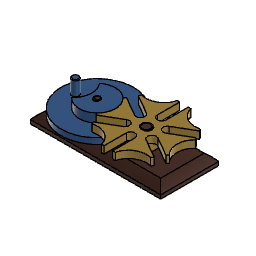
Geneva Mechanism (Autodesk Fusion 360 design; units mm, degrees)
Autodesk Fusion 360 part; units mm, degrees
sketch "Sketch1" plane through (0, 0, 0) normal (0, 0, 1) x (1, 0, 0)
  line L0 (0, 0) -> (180, 0)
  line L1 (180, 0) -> (180, 80)
  line L2 (180, 80) -> (0, 80)
  line L3 (0, 80) -> (0, 0)
  line L4 (90, 80) -> (90, 0) construction
  line L5 (0, 40) -> (180, 40) construction
  circle A0 centre (52.5, 40) radius 7.5
  line L6 (60, 40) -> (90, 40)
  circle A1 centre (120, 40) radius 7.5
  circle A2 centre (52.5, 40) radius 50
  circle A3 centre (52.5, 40) radius 25
  line L7 (70, 68.8675) -> (70, 11.1325) construction
  line L8 (70, 11.1325) -> (120, -17.735) construction
  line L9 (120, -17.735) -> (170, 11.1325) construction
  line L10 (170, 11.1325) -> (170, 68.8675) construction
  line L11 (170, 68.8675) -> (120, 97.735) construction
  line L12 (120, 97.735) -> (70, 68.8675) construction
  circle A4 centre (87.5, 40) radius 25
  line L13 (120, 40) -> (70, 11.1325) construction
  line L14 (98.3234, 34.4132) -> (67, 16.3286)
  line L15 (104.3234, 24.0209) -> (73, 5.9363)
  line L16 (120, 40) -> (70, 68.8675) construction
  line L17 (104.3234, 55.9791) -> (73, 74.0637)
  line L18 (67, 63.6714) -> (98.3234, 45.5868)
  line L19 (170, 40) -> (187.5, 40) construction
  line L20 (120, 40) -> (145, -3.3013) construction
  line L21 (145, -3.3013) -> (153.75, -18.4567) construction
  line L22 (120, 40) -> (145, 83.3013) construction
  line L23 (145, 83.3013) -> (153.75, 98.4567) construction
  circle A5 centre (187.5, 40) radius 25
  circle A6 centre (153.75, 98.4567) radius 25
  circle A7 centre (153.75, -18.4567) radius 25
  line L24 (52.5, 40) -> (70, 11.1325) construction
  circle A8 centre (85, 40) radius 5
  line L25 (95, -3.3013) -> (86.25, -18.4567) construction
  circle A9 centre (86.25, -18.4567) radius 25
  line L26 (120, 40) -> (95, 83.3013) construction
  line L27 (95, 83.3013) -> (86.25, 98.4567) construction
  circle A10 centre (86.25, 98.4567) radius 25
  arc A11 (67, 16.3286) -> (73, 5.9363) centre (70, 11.1325) ccw
  arc A12 (104.3234, 24.0209) -> (98.3234, 34.4132) centre (101.3234, 29.2171) ccw
  arc A13 (73, 74.0637) -> (67, 63.6714) centre (70, 68.8675) ccw
  arc A14 (98.3234, 45.5868) -> (104.3234, 55.9791) centre (101.3234, 50.7829) ccw
  circle A15 centre (120, 97.735) radius 6
  circle A16 centre (170, 68.8675) radius 6
  circle A17 centre (170, 11.1325) radius 6
  circle A18 centre (138.6685, 29.2222) radius 6
  circle A19 centre (138.6767, 50.783) radius 6
  circle A20 centre (120, 61.566) radius 6
  line L28 (120, 67.566) -> (120, 97.735) construction
  line L29 (143.8729, 53.783) -> (170, 68.8675) construction
  line L30 (120, 40) -> (126.4952, 36.25) construction
  line L31 (143.8644, 26.2219) -> (170, 11.1325) construction
  line L32 (70, 22.1464) -> (71.7692, 19.0821)
  line L33 (79.5384, 5.6255) -> (77.7692, 8.6898)
  line L34 (114, 18.434) -> (114, -17.735)
  line L35 (126, 18.434) -> (126, -17.735)
  line L36 (120, 40) -> (120, 24.434) construction
  line L37 (120, 12.434) -> (120, -17.735) construction
  arc A21 (126, 18.434) -> (114, 18.434) centre (120, 18.434) ccw
  arc A22 (114, -17.735) -> (126, -17.735) centre (120, -17.735) ccw
  line L38 (173.0001, 16.3286) -> (141.6685, 34.4183)
  line L39 (135.6684, 24.0261) -> (166.9999, 5.9364)
  line L40 (167, 74.0637) -> (135.6767, 55.9792)
  line L41 (173, 63.6714) -> (141.6767, 45.5868)
  line L42 (114, 97.735) -> (114, 61.566)
  line L43 (126, 97.735) -> (126, 61.566)
  line L44 (110.4616, -12.2281) -> (114, -12.2281)
  line L45 (129.5384, -12.2281) -> (126, -12.2281)
  line L46 (160.4616, 5.6255) -> (162.2309, 8.6899)
  line L47 (170, 22.1464) -> (168.2308, 19.0822)
  line L48 (170, 57.8536) -> (168.2308, 60.9179)
  line L49 (160.4616, 74.3745) -> (162.2308, 71.3102)
  line L50 (129.5384, 92.2281) -> (126, 92.2281)
  line L51 (110.4616, 92.2281) -> (114, 92.2281)
  line L52 (70, 57.8536) -> (71.7692, 60.9179)
  line L53 (79.5384, 74.3745) -> (77.7692, 71.3102)
  circle A23 centre (120, 40) radius 12.5
  circle A24 centre (52.5, 40) radius 5
  circle A25 centre (52.5, 40) radius 12.5
  circle A26 centre (52.5, 40) radius 4
  circle A27 centre (120, 40) radius 6.5
  point P0 (120, 40)
  point P1 (70, 57.8536)
  point P2 (70, 40)
  point P3 (77.5, 40)
  point P4 (102.5, 40)
  point P5 (65.46, 18.6215)
  dimension "d2" = 30
  dimension "d4" = 30
  dimension "d5" = 100
  dimension "d6" = 50
  dimension "d8" = 50
  dimension "d10" = 180
  dimension "d11" = 80
  dimension "d15" = 12
  dimension "d19" = 17.5
  dimension "d26" = 7.4891
  dimension "d27" = 10
  dimension "d28" = 7.5
  dimension "d48" = 25
  dimension "d61" = -1
  dimension "d62" = -1
  constraint horizontal L0
  constraint vertical L1
  constraint horizontal L2
  constraint vertical L3
  constraint coincident L0.start L3.end
  constraint midpoint L2 L4.start
  constraint midpoint L0 L4.end
  constraint midpoint L3 L5.start
  constraint midpoint L1 L5.end
  constraint coincident L5 A0.centre
  constraint coincident L5 L6.start
  constraint coincident A0 L6.start
  constraint midpoint L5 L6.end
  constraint perpendicular L4 L6
  constraint coincident L5 P0
  constraint concentric A0 A2
  constraint concentric A2 A3
  constraint coincident P0 A1.centre
  constraint parallel L4 L7
  constraint coincident L5 A4.centre
  constraint coincident A3 P1
  constraint coincident L7 P1
  constraint midpoint L7 P2
  constraint coincident L5 P3
  constraint coincident A3 P3
  constraint coincident A4 P1
  constraint coincident A2 P4
  constraint coincident L5 P4
  constraint coincident L7.end L8.start
  constraint coincident L13 A12.centre
  constraint coincident A2 A12.centre
  constraint tangent L14 A11
  constraint tangent L15 A11
  constraint tangent L14 A12
  constraint tangent L15 A12
  constraint coincident L7.start L12.end
  constraint coincident L16 A14.centre
  constraint coincident A2 A14.centre
  constraint parallel L16 L17
  constraint tangent L18 A14
  constraint tangent L18 A13
  constraint tangent L17 A13
  constraint tangent L17 A14
  constraint midpoint L10 L19.start
  constraint perpendicular L10 L19
  constraint midpoint L9 L20.end
  constraint perpendicular L9 L21
  constraint midpoint L11 L22.end
  constraint perpendicular L11 L23
  constraint coincident L19.end A5.centre
  constraint coincident L23.end A6.centre
  constraint coincident L21.end A7.centre
  constraint coincident A0.centre A2.centre
  constraint coincident L24 P5
  constraint coincident A3 P5
  constraint coincident L5 A8.centre
  constraint midpoint L8 L25.start
  constraint perpendicular L8 L25
  constraint coincident L25.end A9.centre
  constraint midpoint L12 L26.end
  constraint perpendicular L12 L27
  constraint coincident L27.end A10.centre
  constraint coincident L11.end L12.start
  constraint coincident L10.end L11.start
  constraint coincident L8.end L9.start
  constraint coincident L9.end L10.start
  constraint coincident A20 L28.start
  constraint coincident A19 L29.start
  constraint coincident A1 L30.end
  constraint collinear L30 L31
  constraint coincident A3 L32.start
  constraint coincident A4 L32.start
  constraint coincident L14 L32.end
  constraint perpendicular L14 L32
  constraint coincident A9 L33.start
  constraint coincident L8 L33.start
  constraint coincident L15 L33.end
  constraint perpendicular L15 L33
  constraint tangent L34 A22
  constraint tangent L35 A22
  constraint tangent L34 A21
  constraint tangent L35 A21
  constraint coincident L36.end A21
  constraint collinear L36 L37
  constraint coincident A18 L31.start
  constraint coincident A17 L38.start
  constraint coincident A18 L38.end
  constraint tangent A18 L38
  constraint coincident A18 L39.start
  constraint coincident A17 L39.end
  constraint tangent A17 L39
  constraint coincident A16 L40.start
  constraint coincident A19 L40.end
  constraint tangent A19 L40
  constraint coincident A16 L41.start
  constraint coincident A19 L41.end
  constraint tangent A19 L41
  constraint coincident A15 L42.start
  constraint coincident A20 L42.end
  constraint tangent A20 L42
  constraint coincident A15 L43.start
  constraint coincident A20 L43.end
  constraint tangent A20 L43
  constraint tangent A15 L42
  constraint tangent A15 L43
  constraint tangent A16 L40
  constraint tangent A16 L41
  constraint tangent A17 L38
  constraint tangent A18 L39
  constraint coincident A9 L44.start
  constraint coincident L8 L44.start
  constraint coincident L34 L44.end
  constraint perpendicular L34 L44
  constraint coincident L9 L45.start
  constraint coincident A7 L45.start
  constraint coincident L35 L45.end
  constraint perpendicular L35 L45
  constraint coincident A7 L46.start
  constraint coincident L9 L46.start
  constraint coincident L39 L46.end
  constraint perpendicular L39 L46
  constraint coincident A5 L47.start
  constraint coincident L10 L47.start
  constraint coincident L38 L47.end
  constraint perpendicular L38 L47
  constraint coincident L10 L48.start
  constraint coincident A5 L48.start
  constraint coincident L41 L48.end
  constraint perpendicular L41 L48
  constraint coincident A6 L49.start
  constraint coincident L11 L49.start
  constraint coincident L40 L49.end
  constraint perpendicular L40 L49
  constraint coincident A6 L50.start
  constraint coincident L11 L50.start
  constraint coincident L43 L50.end
  constraint perpendicular L43 L50
  constraint coincident L12 L51.start
  constraint coincident A10 L51.start
  constraint coincident L42 L51.end
  constraint perpendicular L42 L51
  constraint coincident P1 L52.start
  constraint coincident L18 L52.end
  constraint perpendicular L18 L52
  constraint coincident L12 L53.start
  constraint coincident A10 L53.start
  constraint coincident L17 L53.end
  constraint perpendicular L17 L53
  constraint concentric A2 A24
  constraint concentric A0 A25
  measures "d2" distance of L6.start L6.end
  measures "d4" distance of L6.end P0
  measures "d5" diameter of A2
  measures "d6" diameter of A3
  measures "d8" diameter of A4
  measures "d10" distance of L0.start L0.end
  measures "d11" distance of L0.start L2.end
  measures "d15" diameter of A11
  measures "d19" distance of A0.centre P2
  measures "d26" vertical distance of L7.end P5
  measures "d27" diameter of A8
  measures "d28" distance of P3 A8.centre
  measures "d48" diameter of A23
extrude "Extrude4" add sketch "Sketch1" along normal blind 20 contours A3 A4 A25 | A4 A25 | A0 | L6 A8 | L6 A8 makes body 1 at (69.1068, 21.3127, 13.3333) makes body 2 at (89.9752, 40.4978, 13.3333)
extrude "Extrude1" add sketch "Sketch1" along normal blind 10 separate body contours A2 A4 L15 A9 L33 | L0 L2 A2 A4 A5 A6 A7 A9 A10 A18 A19 A20 L34 L35 A21 L38 L39 L40 L41 L42 L43 L46 L47 L48 L49 A23 | L0 A9 L34 L44 | A2 A4 L17 A10 L53 | A2 A4 L15 | A2 A4 L15 L17 A12 A14 A23 | L2 A10 L42 L51 | L0 A7 L35 L45 | A4 A23 | A4 A23 | A4 L14 L32 | A2 A3 A4 L14 L18 A12 A14 | A2 A4 L17 | L2 A6 L43 L50 | A4 L18 L52 | L6 A8 | L6 A8 makes body 3
extrude "Extrude2" add sketch "Sketch1" against normal blind 12 contours A4 A23 | A4 A23 bodies 3
copy_body "Body->Comp1" bodies 3 removing the originals makes body 4 in component "Hexagon"
extrude "Extrude3" add sketch "Sketch1" along normal blind 10 separate body contours L0 L2 A2 A3 L14 L15 L17 L18 A9 A10 A11 A13 L32 L33 L52 L53 | L0 A2 A9 | L0 A2 A9 | L0 A2 A9 | L2 A2 A10 | A2 A4 L15 A9 L33 | L2 A2 A10 | L2 A2 A10 | A4 L14 L15 A11 | A2 A4 L17 A10 L53 | A2 A4 L15 | A2 A4 L14 L15 A12 | A4 L17 L18 A13 | A4 L14 L32 | A2 A3 A4 L14 L18 A12 A14 | A2 A4 L17 | A2 A4 L17 L18 A14 | L6 A3 A4 A25 | A3 A4 A25 | A4 L18 L52 | L6 A3 A4 A25 | A4 A25 | L6 A4 A25 | L6 A4 A25 | A0 | L6 A8 | L6 A8 picked at (40.1327, -1.2898) picked at (81.6151, 3.9769) picked at (71.9676, -3.565) picked at (40.1327, 81.2898) picked at (71.9676, 83.565) picked at (81.6151, 76.0231) makes body 5
combine "Combine1" operation add target body 1 tool bodies 2 5
extrude "Extrude5" add sketch "Sketch1" against normal blind 2 contours A4 A25 | L6 A4 A25 | L6 A4 A25 bodies 1
copy_body "Body->Comp2" bodies 1 removing the originals makes body 6 in component "Circle"
extrude "Extrude6" add sketch "Sketch1" along normal blind 24 separate body contours A26 | A27 makes body 7 at (56.495, 39.8006, 16) makes body 8 at (126.4919, 39.676, 16)
extrude "Extrude7" add sketch "Sketch1" against normal blind 15 contours L0 L2 L3 A2 | L0 L2 A2 A3 L14 L15 L17 L18 A9 A10 A11 A13 L32 L33 L52 L53 | L0 A2 A9 | L0 A2 A9 | A2 A4 L15 A9 L33 | L2 A2 A10 | L0 L2 A2 A4 A5 A6 A7 A9 A10 A18 A19 A20 L34 L35 A21 L38 L39 L40 L41 L42 L43 L46 L47 L48 L49 A23 | A4 L14 L15 A11 | L2 A2 A10 | A2 A4 L17 A10 L53 | L0 L34 L35 A21 | A2 A4 L15 | A2 A4 L15 L17 A12 A14 A23 | A2 A4 L14 L15 A12 | A4 L17 L18 A13 | A2 L15 A12 | A4 A23 | A1 | A4 A23 | A4 L14 L32 | A2 A3 A4 L14 L18 A12 A14 | L2 A20 L42 L43 | A2 A4 L17 | A2 A4 L17 L18 A14 | L0 A7 | L6 A3 A4 A25 | A3 A4 A25 | A20 | A2 L17 A14 | A4 L18 L52 | L0 L1 A5 A7 A17 L38 L39 L46 L47 | L6 A3 A4 A25 | A4 A25 | L6 A4 A25 | L2 A6 | A17 A18 L38 L39 | L6 A4 A25 | L1 L2 A5 A6 A16 L40 L41 L48 L49 | L1 A5 | A18 | A17 | A16 A19 L40 L41 | A16 | A19 | A0 | L6 A8 | L6 A8 | A24 | A26 | A27 picked at (81.6151, 3.9769) picked at (90.189, 0.6547) picked at (81.6151, 76.0231) picked at (95.4497, 79.3605) picked at (155.593, 3.5272) picked at (158.6135, 79.3853) picked at (177.4057, 46.5949) bodies 7 8
copy_body "Body->Comp3" bodies 7 removing the originals makes body 9 in component "Base"
move_body "Move1" bodies 9 to x (1, 0, 0) y (0, 1, 0) z (0, 0, 1) at (0, 0, 15) in component "Base"
move_body "Move1'" bodies 6 to x (-1, 0, 0) y (0, -1, 0) z (0, 0, 1) at (105, 80, 0) in component "Circle"
fillet "Fillet1" radius 10 tangency weight 0.1 4 edges at (0, 40, 15) (90, 0, 15) (90, 80, 15) (180, 40, 15) on bodies 9 in component "Base"
extrude "Extrude1'" cut 1 faces at (115.1859, 39.9202, 39) faces seen with x (1, 0, 0) y (0, 1, 0) z (0, 0, 1) at (0.5396, -1.5466, -27.0198) along direction (0, 0, -1) blind 2 on bodies 9 bodies 4 in component "Hexagon"
extrude "Extrude1''" cut 1 faces at (115.1859, 39.9202, 39) along direction (0, 0, -1) blind 2 on bodies 9 bodies 9 in component "Base"
extrude "Extrude1'''" cut 1 faces at (51.2702, 39.8013, 39) faces seen with x (1, 0, 0) y (0, 1, 0) z (0, 0, 1) at (0.5396, -1.5466, -17.0198) along direction (0, 0, -1) blind 2 on bodies 9 bodies 6 in component "Circle"
extrude "Extrude2'" cut 1 faces at (51.2702, 39.8013, 39) along direction (0, 0, -1) blind 2 on bodies 9 bodies 9 in component "Base"
fillet "Fillet2" radius 1 2 edges at (113.9399, 42.3505, 37) (48.7707, 41.4465, 37) on bodies 9 in component "Base"
extrude "Extrude2''" add 1 faces at (18.4074, 40.955, 20) along direction (0, 0, 1) blind 8 on bodies 6 bodies 6 in component "Circle"
fillet "Fillet2'" radius 1 1 edges at (24.6616, 41.8081, 28) on bodies 6 in component "Circle"
extrude "Extrude3'" cut 1 faces at (22.1872, 57.0019, 10) along direction (0, 0, -1) blind 2 on bodies 6 bodies 6 in component "Circle"
extrude "Extrude4'" add 1 faces at (41.7411, 40.9936, -2) along direction (0, 0, 1) blind 2 on bodies 6 bodies 6 in component "Circle"
extrude "Extrude5'" cut 1 faces at (41.7411, 40.9936, -2) along direction (0, 0, 1) blind 3 on bodies 6 bodies 6 in component "Circle"
extrude "Extrude6'" add 1 faces at (41.7411, 40.9936, 1) along direction (0, 0, -1) blind 1 on bodies 6 bodies 6 in component "Circle"
extrude "Extrude3''" add sketch "Sketch1" along normal blind 15.8259 contours A4 A25 | L6 A4 A25 | L6 A4 A25 | A0 sketch seen with x (1, 0, 0) y (0, 1, 0) z (0, 0, 1) at (0, 0, 1.1741) bodies 9 in component "Base"
sketch "Hexagon detail" plane through (0, 0, 10) normal (0, 0, 1) x (-1, 0, 0) in component "Hexagon"
  arc A0 (-116.4789, -33.3779) -> (-126.8764, -37.0058) centre (-120.5396, -38.4534) ccw
  arc A1 (-126.8764, -37.0058) -> (-116.4789, -33.3779) centre (-120, -40) ccw
  arc A2 (-79.5384, -74.3745) -> (-110.4616, -92.2281) centre (-86.25, -98.4567) ccw
  line L0 (-79.5384, -74.3745) -> (-77.7692, -71.3102)
  line L1 (-77.7692, -71.3102) -> (-104.3234, -55.9791)
  arc A3 (-98.3234, -45.5868) -> (-104.3234, -55.9791) centre (-101.3234, -50.7829) ccw
  line L2 (-98.3234, -45.5868) -> (-71.7692, -60.9179)
  line L3 (-71.7692, -60.9179) -> (-70, -57.8536)
  arc A4 (-70, -22.1464) -> (-70, -57.8536) centre (-52.5, -40) ccw
  line L4 (-70, -22.1464) -> (-71.7692, -19.0821)
  line L5 (-71.7692, -19.0821) -> (-98.3234, -34.4132)
  arc A5 (-104.3234, -24.0209) -> (-98.3234, -34.4132) centre (-101.3234, -29.2171) ccw
  line L6 (-104.3234, -24.0209) -> (-77.7692, -8.6898)
  line L7 (-77.7692, -8.6898) -> (-79.5384, -5.6255)
  arc A6 (-110.4616, 12.2281) -> (-79.5384, -5.6255) centre (-86.25, 18.4567) ccw
  line L8 (-110.4616, 12.2281) -> (-114, 12.2281)
  line L9 (-114, 12.2281) -> (-114, -18.434)
  arc A7 (-126, -18.434) -> (-114, -18.434) centre (-120, -18.434) ccw
  line L10 (-126, -18.434) -> (-126, 12.2281)
  line L11 (-126, 12.2281) -> (-129.5384, 12.2281)
  arc A8 (-160.4616, -5.6255) -> (-129.5384, 12.2281) centre (-153.75, 18.4567) ccw
  line L12 (-160.4616, -5.6255) -> (-162.2309, -8.6899)
  line L13 (-162.2309, -8.6899) -> (-135.6684, -24.0261)
  arc A9 (-141.6685, -34.4183) -> (-135.6684, -24.0261) centre (-138.6685, -29.2222) ccw
  line L14 (-141.6685, -34.4183) -> (-168.2308, -19.0822)
  line L15 (-168.2308, -19.0822) -> (-170, -22.1464)
  arc A10 (-170, -57.8536) -> (-170, -22.1464) centre (-187.5, -40) ccw
  line L16 (-170, -57.8536) -> (-168.2308, -60.9179)
  line L17 (-168.2308, -60.9179) -> (-141.6767, -45.5868)
  arc A11 (-135.6767, -55.9792) -> (-141.6767, -45.5868) centre (-138.6767, -50.783) ccw
  line L18 (-135.6767, -55.9792) -> (-162.2308, -71.3102)
  line L19 (-162.2308, -71.3102) -> (-160.4616, -74.3745)
  arc A12 (-129.5384, -92.2281) -> (-160.4616, -74.3745) centre (-153.75, -98.4567) ccw
  line L20 (-129.5384, -92.2281) -> (-126, -92.2281)
  line L21 (-126, -92.2281) -> (-126, -61.566)
  arc A13 (-114, -61.566) -> (-126, -61.566) centre (-120, -61.566) ccw
  line L22 (-114, -61.566) -> (-114, -92.2281)
  line L23 (-114, -92.2281) -> (-110.4616, -92.2281)
  circle A14 centre (-120, -40) radius 7.5
  circle A15 centre (-120, -40) radius 6.8
  dimension "d103" = -0.7
  constraint concentric A1 A14
extrude "Extrude3'''" add sketch "Hexagon detail" against normal blind 22 contours A1 A14 bodies 4 in component "Hexagon"
extrude "Extrude2'''" add sketch "Hexagon detail" against normal blind 22 contours A1 A14 bodies 4 in component "Hexagon"
sketch "Circle detail" plane through (0, 0, 20) normal (0, 0, 1) x (-1, 0, 0) in component "Circle"
  arc A0 (-50.3659, -35.4783) -> (-56.9838, -37.7874) centre (-53.0396, -38.4534) ccw
  arc A1 (-56.9838, -37.7874) -> (-50.3659, -35.4783) centre (-52.5, -40) ccw
  arc A2 (-35, -22.1464) -> (-35, -57.8536) centre (-52.5, -40) ccw
  arc A3 (-35, -22.1464) -> (-35, -57.8536) centre (-17.5, -40) ccw
  circle A4 centre (-52.5, -40) radius 5
  circle A5 centre (-52.5, -40) radius 4.3
  dimension "d106" = -0.7
  constraint concentric A1 A4
extrude "Extrude8" add sketch "Circle detail" against normal blind 20 contours A1 A4 bodies 6 in component "Circle"
extrude "Extrude7'" add sketch "Circle detail" against normal blind 20 contours A1 A4 bodies 6 in component "Circle"
sketch "Sketch2" plane through (0, 0, 0) normal (0, 1, 0) x (1, 0, 0)
component "Hexagon" placed x (1, 0, 0) y (0, 1, 0) z (0, 0, 1) at (0, 0, 25.8259)
component "Circle" placed x (0.997981, -0.063511, 0) y (0.063511, 0.997981, 0) z (0, 0, 1) at (-2.4344, 3.4151, 15.8259)
component "Base" placed x (1, 0, 0) y (0, 1, 0) z (0, 0, 1) at (0, 0, -1.1741)
named bodies: "Hexagon", "Circle", "Base"
